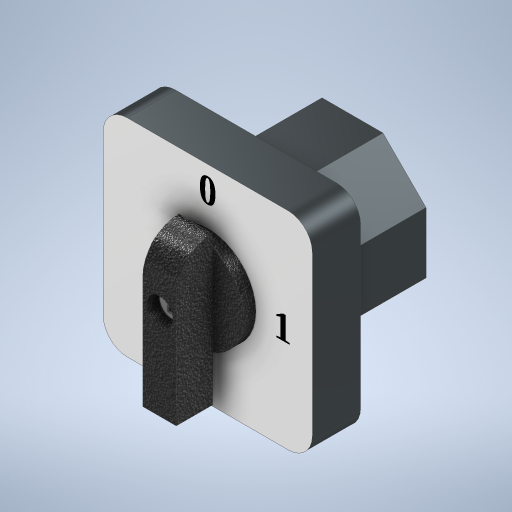
# Autodesk Inventor part: gabaritna_sklopka
Saved by Autodesk Inventor 2023 (Build 270158000, 158)
## iProperties
Created: 2022-07-08
Part Number: gabaritna_sklopka
Material: Generic
Document SubType Name: Modeling
Designer: User
Density: 1 g/cm^3
Appearance: Default
Author: User
Autodesk Inventor part; units mm, degrees
ref_plane "YZ Plane" through (0, 0, 0) normal (1, 0, 0) x (0, 1, 0)
ref_plane "XZ Plane" through (0, 0, 0) normal (0, 1, 0) x (-1, 0, 0)
ref_plane "XY Plane" through (0, 0, 0) normal (0, 0, 1) x (1, 0, 0)
sketch "Sketch1" plane through (0, 0, 0) normal (0, 0, 1) x (1, 0, 0)
  line L0 (-12.6252, -30.48) -> (-30.48, -12.6252)
  line L1 (-30.48, -12.6252) -> (-30.48, 12.6252)
  line L2 (-30.48, 12.6252) -> (-12.6252, 30.48)
  line L3 (-12.6252, 30.48) -> (12.6252, 30.48)
  line L4 (12.6252, 30.48) -> (30.48, 12.6252)
  line L5 (30.48, 12.6252) -> (30.48, -12.6252)
  line L6 (30.48, -12.6252) -> (12.6252, -30.48)
  line L7 (12.6252, -30.48) -> (-12.6252, -30.48)
  circle A0 centre (0, 0) radius 30.48
  line L8 (28.3719, -11.1385) -> (12.1858, -27.9381)
  line L9 (12.1858, -27.9381) -> (-11.1385, -28.3719)
  line L10 (-11.1385, -28.3719) -> (-27.9381, -12.1858)
  line L11 (-27.9381, -12.1858) -> (-28.3719, 11.1385)
  line L12 (-28.3719, 11.1385) -> (-12.1858, 27.9381)
  line L13 (-12.1858, 27.9381) -> (11.1385, 28.3719)
  line L14 (11.1385, 28.3719) -> (27.9381, 12.1858)
  line L15 (27.9381, 12.1858) -> (28.3719, -11.1385)
  point P0 (0, 0)
  point P1 (0, 30.48)
  dimension "d50" = 60.96
  dimension "d54" = 30.48
  constraints: 32 end point, 2 coincident, 1 midpoint, 37 other
  measures "d54" distance of point (0, 30.48) point (0, 0)
extrude "Extrusion1" add sketch "Sketch1" along normal blind 40
sketch "Sketch2" plane through (0, 0, 40) normal (0, 0, 1) x (1, 0, 0)
  line L0 (-43.3633, -42.9193) -> (43.3633, -42.9193)
  line L1 (43.3633, -42.9193) -> (43.3633, 42.9193)
  line L2 (43.3633, 42.9193) -> (-43.3633, 42.9193)
  line L3 (-43.3633, 42.9193) -> (-43.3633, -42.9193)
  line L4 (-43.3633, -42.9193) -> (43.3633, 42.9193) construction
  line L5 (43.3633, -42.9193) -> (-43.3633, 42.9193) construction
  point P0 (0, 0)
  constraints: 12 end point, 2 midpoint, 2 parallel, 1 horizontal, 1 perpendicular
extrude "Extrusion2" add sketch "Sketch2" along normal blind 20
fillet "Fillet1" radius 10 4 edges at (43.3633, 42.9193, 50) (43.3633, -42.9193, 50) (-43.3633, 42.9193, 50) (-43.3633, -42.9193, 50)
sketch "Sketch3" plane through (0, 0, 60) normal (0, 0, 1) x (1, 0, 0)
  circle A0 centre (0, 0) radius 19.9292
  constraints: 1 centre point, 1 coincident
extrude "Extrusion3" add sketch "Sketch3" along normal blind 5
sketch "Sketch4" plane through (0, 0, 65) normal (0, 0, 1) x (1, 0, 0)
  line L0 (6.9511, -37.5125) -> (-6.9511, -37.5125)
  line L1 (-6.9511, -37.5125) -> (-6.9511, 24.1539)
  line L2 (-6.9511, 24.1539) -> (6.9511, 24.1539)
  line L3 (6.9511, 24.1539) -> (6.9511, -37.5125)
  line L4 (6.9511, -37.5125) -> (-6.9511, 24.1539) construction
  line L5 (-6.9511, -37.5125) -> (6.9511, 24.1539) construction
  point P0 (0, 0)
  point P1 (0, -6.6793)
  constraints: 12 end point, 2 midpoint, 2 parallel, 1 horizontal, 1 perpendicular
extrude "Extrusion4" add sketch "Sketch4" along normal blind 15
fillet "Fillet2" radius 15 1 edges at (0, 24.1539, 80)
sketch "Sketch5" plane through (0, 0, 80) normal (0, 0, 1) x (1, 0, 0)
  circle A0 centre (0, 0) radius 5.639
  constraints: 1 centre point, 1 coincident
extrude "Extrusion5" cut sketch "Sketch5" against normal blind 20
sketch "Sketch6" plane through (0, 0, 60) normal (0, 0, 1) x (1, 0, 0)
  circle A0 centre (0, 0) radius 5.639 projected
  circle A1 centre (0, 0) radius 5.08
  dimension "d13" = 10.16
  constraints: 1 centre point, 1 coincident
  measures "d13" diameter of A1
extrude "Extrusion6" add sketch "Sketch6" along normal blind 15 contours A1
sketch "Sketch7" plane through (0, 0, 75) normal (0, 0, 1) x (1, 0, 0)
  line L0 (1.4769, -3.2223) -> (-1.4769, -3.2223)
  line L1 (-1.4769, -3.2223) -> (-1.4769, 3.2223)
  line L2 (-1.4769, 3.2223) -> (1.4769, 3.2223)
  line L3 (1.4769, 3.2223) -> (1.4769, -3.2223)
  circle A0 centre (0, 0) radius 5.639 projected
  line L4 (1.4769, -3.2223) -> (-1.4769, 3.2223) construction
  line L5 (-1.4769, -3.2223) -> (1.4769, 3.2223) construction
  constraints: 12 end point, 2 midpoint, 2 parallel, 1 horizontal, 1 perpendicular
extrude "Extrusion7" cut sketch "Sketch7" against normal blind 5 contours L0 L1 L2 L3
sketch "Sketch8" plane through (0, 0, 60) normal (0, 0, 1) x (1, 0, 0)
  line L0 (-9.528, 62.156) -> (8.3554, 62.156) construction
  line L1 (8.3554, 62.156) -> (8.3554, 44.2726) construction
  line L2 (8.3554, 44.2726) -> (-9.528, 44.2726) construction
  line L3 (-9.528, 44.2726) -> (-9.528, 62.156) construction
  line L4 (44.1222, 9.3815) -> (61.4167, 9.3815) construction
  line L5 (61.4167, 9.3815) -> (61.4167, -7.913) construction
  line L6 (61.4167, -7.913) -> (44.1222, -7.913) construction
  line L7 (44.1222, -7.913) -> (44.1222, 9.3815) construction
  point P0 (0, 0)
  constraints: 4 other
decal "Decal1"
decal "Decal2"
sketch "Sketch9" plane through (-30.48, 12.6252, 0) normal (-1, 0, 0) x (0, -1, 0)
  point P0 (12.6252, 0)
sketch "Sketch10" plane through (0, 0, 60) normal (0, 0, 1) x (1, 0, 0)
  line L0 (-5.7001, 39.3416) -> (5.3375, 39.3416) construction
  line L1 (5.3375, 39.3416) -> (5.3375, 28.3041) construction
  line L2 (5.3375, 28.3041) -> (-5.7001, 28.3041) construction
  line L3 (-5.7001, 28.3041) -> (-5.7001, 39.3416) construction
  line L4 (25.3709, 6.0354) -> (36.3058, 6.0354) construction
  line L5 (36.3058, 6.0354) -> (36.3058, -4.8995) construction
  line L6 (36.3058, -4.8995) -> (25.3709, -4.8995) construction
  line L7 (25.3709, -4.8995) -> (25.3709, 6.0354) construction
  point P0 (0, 0)
  constraints: 4 other
decal "Decal3"
decal "Decal4"
body "Solid1"
